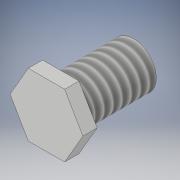
# Autodesk Inventor part: Pedal Bar Bolt
Saved by Autodesk Inventor 2019 (Build 230136000, 136)
## iProperties
Created: 2020-06-01
Part Number: Pedal Bar Bolt
Material: Generic
Document SubType Name: Modeling
Designer: 18186
Density: 1 g/cm^3
Appearance: Default
Author: 18186
Autodesk Inventor part; units mm, degrees
ref_plane "YZ Plane" through (0, 0, 0) normal (1, 0, 0) x (0, 1, 0)
ref_plane "XZ Plane" through (0, 0, 0) normal (0, 1, 0) x (-1, 0, 0)
ref_plane "XY Plane" through (0, 0, 0) normal (0, 0, 1) x (1, 0, 0)
sketch "Sketch1" plane through (0, 0, 0) normal (0, 0, 1) x (1, 0, 0)
  circle A0 centre (0, 0) radius 1.5875
  dimension "d0" = 3.175
  constraints: 1 centre point, 1 coincident
  measures "d0" diameter of A0
extrude "Extrusion1" add sketch "Sketch1" along normal blind 5.08
sketch "Sketch2" plane through (0, 0, 5.08) normal (0, 0, 1) x (1, 0, 0)
  line L0 (2.54, 0) -> (1.27, -2.1997)
  line L1 (1.27, -2.1997) -> (-1.27, -2.1997)
  line L2 (-1.27, -2.1997) -> (-2.54, 0)
  line L3 (-2.54, 0) -> (-1.27, 2.1997)
  line L4 (-1.27, 2.1997) -> (1.27, 2.1997)
  line L5 (1.27, 2.1997) -> (2.54, 0)
  point P0 (0, 0)
  point P1 (0, 0)
  dimension "d5" = 5.08
  constraints: 12 end point, 1 coincident, 13 other
  measures "d5" distance of L0.start L2.end
extrude "Extrusion2" add sketch "Sketch2" along normal blind 1
thread "Thread1" size "5-40 UNC" class "2A" standard "ANSI Unified Screw Threads" full length
body "Solid1"
